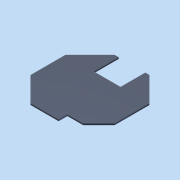
# Autodesk Inventor part: Tant_Exp4_top
Saved by Autodesk Inventor 2014 SP1 (Build 180222100, 222)
## iProperties
Created: 2013-09-02
Part Number: Tant_Exp4_top
Document SubType Name: Modeling
Designer: Robert Davis
Density: 11.37 g/cm^3
Material: Lead
Mass: 119.543 g
Surface Area: 139.396 cm^2
Volume: 10.5139 cm^3
Appearance: Lead
Author: Robert Davis
Autodesk Inventor part; units mm, degrees
ref_plane "YZ Plane" through (0, 0, 0) normal (1, 0, 0) x (0, 1, 0)
ref_plane "XZ Plane" through (0, 0, 0) normal (0, 1, 0) x (-1, 0, 0)
ref_plane "XY Plane" through (0, 0, 0) normal (0, 0, 1) x (1, 0, 0)
sketch "Sketch1" plane through (0, 0, 0) normal (0, 0, 1) x (1, 0, 0)
  line L0 (0, 0) -> (0, 24.8008)
  line L1 (0, 0) -> (23.5103, 0)
  line L2 (-19.7, 47.5) -> (19.7, 47.5)
  line L3 (47.5, 19.7) -> (47.5, -19.7)
  line L4 (19.7, -47.5) -> (-19.7, -47.5)
  line L5 (-47.5, -19.7) -> (-47.5, 19.7)
  line L6 (19.7, 47.5) -> (47.5, 19.7)
  line L7 (47.5, -19.7) -> (19.7, -47.5)
  line L8 (-19.7, -47.5) -> (-47.5, -19.7)
  line L9 (-47.5, 19.7) -> (-19.7, 47.5)
  point P0 (-47.5, 47.5)
  point P1 (47.5, -47.5)
  point P2 (47.5, 47.5)
  point P3 (-47.5, -47.5)
  dimension "d9" = 27.8
  dimension "d10" = 27.8
  dimension "d11" = 27.8
  dimension "d12" = 27.8
  dimension "d13" = 27.8
  dimension "d14" = 27.8
  dimension "d15" = 27.8
  dimension "d16" = 27.8
  dimension "d17" = 95
  dimension "d18" = 95
  constraints: 20 end point, 8 point on line, 2 horizontal, 2 vertical, 1 coincident, 3 other
  measures "d9" distance of L2.end point (47.5, 47.5)
  measures "d10" distance of L3.start point (47.5, 47.5)
  measures "d11" distance of L3.end point (47.5, -47.5)
  measures "d12" distance of L4.start point (47.5, -47.5)
  measures "d13" distance of L4.end point (-47.5, -47.5)
  measures "d14" distance of L5.start point (-47.5, -47.5)
  measures "d15" distance of L5.end point (-47.5, 47.5)
  measures "d16" distance of L2.start point (-47.5, 47.5)
  measures "d17" distance between parallel lines of L4 L2
  measures "d18" distance between parallel lines of L3 L5
extrude "Extrusion1" add sketch "Sketch1" along normal mid plane 1.5748
sketch "Sketch2" plane through (0, 0, 0.7874) normal (0, 0, 1) x (1, 0, 0)
  line L0 (0, 0) -> (0, 42.1348)
  line L1 (-15, 47.5) -> (15, 47.5)
  line L2 (15, 47.5) -> (15, 19.5)
  line L3 (15, 19.5) -> (-15, 19.5)
  line L4 (-15, 19.5) -> (-15, 47.5)
  line L5 (-19.7, 47.5) -> (19.7, 47.5) projected
  dimension "d4" = 30
  dimension "d25" = 28
  constraints: 10 end point, 2 horizontal, 2 vertical, 1 coincident, 1 collinear, 1 other
  measures "d4" distance of L2.end L3.end
  measures "d25" distance of L3.end L1.start
extrude "Extrusion2" cut sketch "Sketch2" against normal through all
sketch "Sketch3" plane through (0, 0, 0.7874) normal (0, 0, 1) x (1, 0, 0)
  line L0 (19.7, -47.5) -> (-19.7, -47.5) projected
  line L1 (12, -47.5) -> (32, -47.5)
  line L2 (32, -47.5) -> (32, -37.5)
  line L3 (32, -37.5) -> (12, -37.5)
  line L4 (12, -37.5) -> (12, -47.5)
  point P0 (0, 0)
  dimension "d19" = 10
  dimension "d21" = 12
  dimension "d24" = 32
  constraints: 8 end point, 2 horizontal, 2 vertical, 1 collinear
  measures "d19" distance of L3.end L1.start
  measures "d21" distance from line of point (0, 0) L4
  measures "d24" distance from line of point (0, 0) L2
extrude "Extrusion3" cut sketch "Sketch3" against normal through all
equation "\"d10\" = d9"
equation "\"d11\" = d9"
equation "\"d12\" = d11"
equation "\"d13\" = d9"
equation "\"d14\" = d13"
equation "\"d15\" = d9"
equation "\"d16\" = d15"
body "Solid1"
